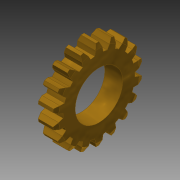
# Autodesk Inventor part: Zahnrad Messing z18
Saved by Autodesk Inventor 2019.3 (Build 233278000, 278)
## iProperties
Category: PARTsolutions
Company: MAEDLER
Created: 2018-08-20
Part Number: Zahnrad Messing z18
Material: Messing, weicher Gelbton, geschweißt
Catalog Web Link: www.cadenas.de
Description: Stzr Messing Ms58-Spur Gears, Brass, Helical Tooth Right Hand, with one-sided hub
Vendor: MAEDLER
Document SubType Name: Modeling
Designer: psadmin
Manufacturer: MAEDLER
Mass: 2.2 g
Surface Area: 3.45567 cm^2
Volume: 0.259692 cm^3
Density: 8.47159 g/cm^3
Appearance: Schweißnaht - Messing
PSOL_IDENT_0: {$CADENAS_DATA\23d-libs\maedler\antriebselemente\stirnzahnraeder\stirnzahnraeder_messing\stzr_messin
PSOL_IDENT_1: g_ms58.prj},204 {VTYP=3D},{NB=Stzr Messing Ms58 26101800},{LINA=Stzr Messing Ms58 26101800},{NN=Stzr
PSOL_IDENT_2: Messing Ms58},{DATE=03.08.2018 09:08:56},{GEOMDATE=26.07.2018 09:15:44},{VERSION=},{LINEID=250},{WB
PSOL_IDENT_3: VAR=},{WBNUMERIC=}  {NB=Stzr Messing Ms58 26101800},{LINA=Stzr Messing Ms58 26101800},{KT=DUMMY},{AR
PSOL_IDENT_4: TNR=26101800},{WST=Messing (Ms58)},{M=0.5},{Z=18},{PDF=PDF Katalogseite},{B1=2.0},{DA=10.00},{D=9.00
PSOL_IDENT_5: },{NL=4},{ND=7},{B=2.00},{MD=0.9},{GEW=2.200}
NN: Stzr Messing Ms58
NT: Spur Gears, Brass, Helical Tooth Right Hand, with one-sided hub
NB: Stzr Messing Ms58 26101800
NBSYN: Stzr Messing Ms58 $ARTNR.
LINA: Stzr Messing Ms58 26101800
ARTNR: 26101800
WST: Messing (Ms58)
M: 0.5
Z: 18
PDF: PDF Katalogseite
B1: 2
DA: 10
D: 9
NL: 4
ND: 7
B: 2
MD: 0.9
GEW: 2.2
SUPPLIER: MAEDLER
ARTICLENO: Stzr Messing Ms58 26101800
BOMINFO: Stzr Messing Ms58 26101800
CREATOR: CADENAS GmbH
Title: Stzr Messing Ms58 26101800
Author: Cadenas PARTsolutions
Comments: Spur Gears, Brass, Helical Tooth Right Hand, with one-sided hub
Autodesk Inventor part; units mm, degrees
ref_plane "YZ Plane" through (0, 0, 0) normal (1, 0, 0) x (0, 1, 0)
ref_plane "XZ Plane" through (0, 0, 0) normal (0, 1, 0) x (-1, 0, 0)
ref_plane "XY Plane" through (0, 0, 0) normal (0, 0, 1) x (1, 0, 0)
sketch "Skizze_1" plane through (0, 0, 0) normal (0, 0, 1) x (1, 0, 0)
  line L0 (6, 0) -> (0, 0)
  line L1 (0, 1) -> (6, 1)
  line L2 (6, 1) -> (6, 3.5)
  line L3 (6, 3.5) -> (2, 3.5)
  line L4 (2, 3.5) -> (2, 4.5)
  line L5 (2, 4.5) -> (1, 7.2475)
  line L6 (1, 7.2475) -> (0, 4.5)
  line L7 (0, 4.5) -> (0, 1)
  constraints: 16 end point
revolve "Revolution1" add sketch "Skizze_1" angle 360 about axis through (6, 0, 0) along (1, 0, 0)
sketch "Skizze_2" plane through (2, 0, 0) normal (1, 0, 0) x (0, 0, -1)
  circle A0 centre (0, 0) radius 15
  arc A1 (-4.9972, 0.1667) -> (-4.9972, -0.1667) centre (0, 0) ccw
  line L0 (-4.9972, -0.1667) -> (-4.4844, -0.3742)
  line L1 (-4.4844, -0.3742) -> (-3.973, -0.4644)
  arc A2 (-3.973, -0.4644) -> (-3.8922, -0.9225) centre (0, 0) ccw
  line L2 (-3.8922, -0.9225) -> (-4.342, -1.1821)
  line L3 (-4.342, -1.1821) -> (-4.7529, -1.5525)
  arc A3 (-4.7529, -1.5525) -> (-4.6388, -1.8658) centre (0, 0) ccw
  line L4 (-4.6388, -1.8658) -> (-4.086, -1.8854)
  line L5 (-4.086, -1.8854) -> (-3.5745, -1.7952)
  arc A4 (-3.5745, -1.7952) -> (-3.342, -2.198) centre (0, 0) ccw
  line L6 (-3.342, -2.198) -> (-3.6758, -2.5959)
  line L7 (-3.6758, -2.5959) -> (-3.9352, -3.0845)
  arc A5 (-3.9352, -3.0845) -> (-3.721, -3.3398) centre (0, 0) ccw
  line L8 (-3.721, -3.3398) -> (-3.1947, -3.1692)
  line L9 (-3.1947, -3.1692) -> (-2.745, -2.9095)
  arc A6 (-2.745, -2.9095) -> (-2.3886, -3.2085) centre (0, 0) ccw
  line L10 (-2.3886, -3.2085) -> (-2.5663, -3.6965)
  line L11 (-2.5663, -3.6965) -> (-2.6429, -4.2444)
  arc A7 (-2.6429, -4.2444) -> (-2.3543, -4.4111) centre (0, 0) ccw
  line L12 (-2.3543, -4.4111) -> (-1.9182, -4.0707)
  line L13 (-1.9182, -4.0707) -> (-1.5843, -3.6729)
  arc A8 (-1.5843, -3.6729) -> (-1.1472, -3.832) centre (0, 0) ccw
  line L14 (-1.1472, -3.832) -> (-1.1472, -4.3513)
  line L15 (-1.1472, -4.3513) -> (-1.0319, -4.8924)
  arc A9 (-1.0319, -4.8924) -> (-0.7036, -4.9502) centre (0, 0) ccw
  line L16 (-0.7036, -4.9502) -> (-0.4102, -4.4813)
  line L17 (-0.4102, -4.4813) -> (-0.2326, -3.9932)
  arc A10 (-0.2326, -3.9932) -> (0.2326, -3.9932) centre (0, 0) ccw
  line L18 (0.2326, -3.9932) -> (0.4102, -4.4813)
  line L19 (0.4102, -4.4813) -> (0.7036, -4.9502)
  arc A11 (0.7036, -4.9502) -> (1.0319, -4.8924) centre (0, 0) ccw
  line L20 (1.0319, -4.8924) -> (1.1472, -4.3513)
  line L21 (1.1472, -4.3513) -> (1.1472, -3.832)
  arc A12 (1.1472, -3.832) -> (1.5843, -3.6729) centre (0, 0) ccw
  line L22 (1.5843, -3.6729) -> (1.9182, -4.0707)
  line L23 (1.9182, -4.0707) -> (2.3543, -4.4111)
  arc A13 (2.3543, -4.4111) -> (2.6429, -4.2444) centre (0, 0) ccw
  line L24 (2.6429, -4.2444) -> (2.5663, -3.6965)
  line L25 (2.5663, -3.6965) -> (2.3886, -3.2085)
  arc A14 (2.3886, -3.2085) -> (2.745, -2.9095) centre (0, 0) ccw
  line L26 (2.745, -2.9095) -> (3.1947, -3.1692)
  line L27 (3.1947, -3.1692) -> (3.721, -3.3398)
  arc A15 (3.721, -3.3398) -> (3.9352, -3.0845) centre (0, 0) ccw
  line L28 (3.9352, -3.0845) -> (3.6758, -2.5959)
  line L29 (3.6758, -2.5959) -> (3.342, -2.198)
  arc A16 (3.342, -2.198) -> (3.5745, -1.7952) centre (0, 0) ccw
  line L30 (3.5745, -1.7952) -> (4.086, -1.8854)
  line L31 (4.086, -1.8854) -> (4.6388, -1.8658)
  arc A17 (4.6388, -1.8658) -> (4.7529, -1.5525) centre (0, 0) ccw
  line L32 (4.7529, -1.5525) -> (4.342, -1.1821)
  line L33 (4.342, -1.1821) -> (3.8922, -0.9225)
  arc A18 (3.8922, -0.9225) -> (3.973, -0.4644) centre (0, 0) ccw
  line L34 (3.973, -0.4644) -> (4.4844, -0.3742)
  line L35 (4.4844, -0.3742) -> (4.9972, -0.1667)
  arc A19 (4.9972, -0.1667) -> (4.9972, 0.1667) centre (0, 0) ccw
  line L36 (4.9972, 0.1667) -> (4.4844, 0.3742)
  line L37 (4.4844, 0.3742) -> (3.973, 0.4644)
  arc A20 (3.973, 0.4644) -> (3.8922, 0.9225) centre (0, 0) ccw
  line L38 (3.8922, 0.9225) -> (4.342, 1.1821)
  line L39 (4.342, 1.1821) -> (4.7529, 1.5525)
  arc A21 (4.7529, 1.5525) -> (4.6388, 1.8658) centre (0, 0) ccw
  line L40 (4.6388, 1.8658) -> (4.086, 1.8854)
  line L41 (4.086, 1.8854) -> (3.5745, 1.7952)
  arc A22 (3.5745, 1.7952) -> (3.342, 2.198) centre (0, 0) ccw
  line L42 (3.342, 2.198) -> (3.6758, 2.5959)
  line L43 (3.6758, 2.5959) -> (3.9352, 3.0845)
  arc A23 (3.9352, 3.0845) -> (3.721, 3.3398) centre (0, 0) ccw
  line L44 (3.721, 3.3398) -> (3.1947, 3.1692)
  line L45 (3.1947, 3.1692) -> (2.745, 2.9095)
  arc A24 (2.745, 2.9095) -> (2.3886, 3.2085) centre (0, 0) ccw
  line L46 (2.3886, 3.2085) -> (2.5663, 3.6965)
  line L47 (2.5663, 3.6965) -> (2.6429, 4.2444)
  arc A25 (2.6429, 4.2444) -> (2.3543, 4.4111) centre (0, 0) ccw
  line L48 (2.3543, 4.4111) -> (1.9182, 4.0707)
  line L49 (1.9182, 4.0707) -> (1.5843, 3.6729)
  arc A26 (1.5843, 3.6729) -> (1.1472, 3.832) centre (0, 0) ccw
  line L50 (1.1472, 3.832) -> (1.1472, 4.3513)
  line L51 (1.1472, 4.3513) -> (1.0319, 4.8924)
  arc A27 (1.0319, 4.8924) -> (0.7036, 4.9502) centre (0, 0) ccw
  line L52 (0.7036, 4.9502) -> (0.4102, 4.4813)
  line L53 (0.4102, 4.4813) -> (0.2326, 3.9932)
  arc A28 (0.2326, 3.9932) -> (-0.2326, 3.9932) centre (0, 0) ccw
  line L54 (-0.2326, 3.9932) -> (-0.4102, 4.4813)
  line L55 (-0.4102, 4.4813) -> (-0.7036, 4.9502)
  arc A29 (-0.7036, 4.9502) -> (-1.0319, 4.8924) centre (0, 0) ccw
  line L56 (-1.0319, 4.8924) -> (-1.1472, 4.3513)
  line L57 (-1.1472, 4.3513) -> (-1.1472, 3.832)
  arc A30 (-1.1472, 3.832) -> (-1.5843, 3.6729) centre (0, 0) ccw
  line L58 (-1.5843, 3.6729) -> (-1.9182, 4.0707)
  line L59 (-1.9182, 4.0707) -> (-2.3543, 4.4111)
  arc A31 (-2.3543, 4.4111) -> (-2.6429, 4.2444) centre (0, 0) ccw
  line L60 (-2.6429, 4.2444) -> (-2.5663, 3.6965)
  line L61 (-2.5663, 3.6965) -> (-2.3886, 3.2085)
  arc A32 (-2.3886, 3.2085) -> (-2.745, 2.9095) centre (0, 0) ccw
  line L62 (-2.745, 2.9095) -> (-3.1947, 3.1692)
  line L63 (-3.1947, 3.1692) -> (-3.721, 3.3398)
  arc A33 (-3.721, 3.3398) -> (-3.9352, 3.0845) centre (0, 0) ccw
  line L64 (-3.9352, 3.0845) -> (-3.6758, 2.5959)
  line L65 (-3.6758, 2.5959) -> (-3.342, 2.198)
  arc A34 (-3.342, 2.198) -> (-3.5745, 1.7952) centre (0, 0) ccw
  line L66 (-3.5745, 1.7952) -> (-4.086, 1.8854)
  line L67 (-4.086, 1.8854) -> (-4.6388, 1.8658)
  arc A35 (-4.6388, 1.8658) -> (-4.7529, 1.5525) centre (0, 0) ccw
  line L68 (-4.7529, 1.5525) -> (-4.342, 1.1821)
  line L69 (-4.342, 1.1821) -> (-3.8922, 0.9225)
  arc A36 (-3.8922, 0.9225) -> (-3.973, 0.4644) centre (0, 0) ccw
  line L70 (-3.973, 0.4644) -> (-4.4844, 0.3742)
  line L71 (-4.4844, 0.3742) -> (-4.9972, 0.1667)
  constraints: 144 end point, 72 point on circle, 37 centre point
extrude "Extrusion1" cut sketch "Skizze_2" along normal mid plane 12
sketch "Skizze3" plane through (6, 0, 0) normal (1, 0, 0) x (0, 0, -1)
  circle A0 centre (0, 0) radius 3.5 projected
extrude "Extrusion2" cut sketch "Skizze3" against normal blind 4
sketch "Skizze4" plane through (0, 0, 0) normal (-1, 0, 0) x (0, 0, 1)
  point P0 (0, 0)
  point P1 (0, 0)
  constraints: 1 coincident
hole "Bohrung1" at (0, 0, 0) direction (1, 0, 0) diameter 5.3 end through all
body "Solid1"
